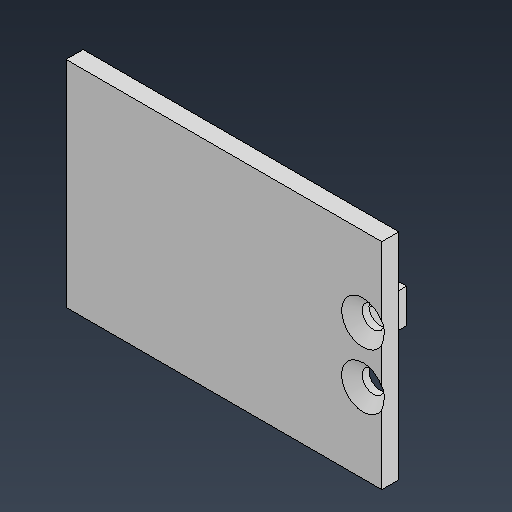
# Autodesk Inventor part: PCB_Holder_Floor
Saved by Autodesk Inventor 2026.2 (Build 302298010, 298A)
## iProperties
Created: 2026-04-05
Part Number: PCB_Holder_Floor
Material: Generic
Document SubType Name: Modeling
Designer: szymo
Density: 1 g/cm^3
Appearance: Default
Author: szymo
Autodesk Inventor part; units mm, degrees
ref_plane "YZ Plane" through (0, 0, 0) normal (1, 0, 0) x (0, 1, 0)
ref_plane "XZ Plane" through (0, 0, 0) normal (0, 1, 0) x (-1, 0, 0)
ref_plane "XY Plane" through (0, 0, 0) normal (0, 0, 1) x (1, 0, 0)
sketch "Sketch1" plane through (0, 0, 0) normal (0, 0, 1) x (1, 0, 0)
  line L0 (-1.35, 35.9569) -> (-38.25, 35.9569)
  line L1 (-38.25, 35.9569) -> (-38.25, 22.861)
  line L2 (-38.25, 22.861) -> (-1.35, 22.861)
  line L3 (-1.35, 22.861) -> (-1.35, 35.9569)
  line L4 (-5.95, 27.409) -> (-11.45, 27.409)
  line L5 (-11.45, 27.409) -> (-11.45, 31.409)
  line L6 (-11.45, 31.409) -> (-5.95, 31.409)
  line L7 (-5.95, 31.409) -> (-5.95, 27.409)
  line L8 (-28.15, 27.409) -> (-33.65, 27.409)
  line L9 (-33.65, 27.409) -> (-33.65, 31.409)
  line L10 (-33.65, 31.409) -> (-28.15, 31.409)
  line L11 (-28.15, 31.409) -> (-28.15, 27.409)
  line L12 (-1.35, 22.861) -> (-1.35, 16.861)
  line L13 (-1.35, 16.861) -> (-38.25, 16.861)
  line L14 (-38.25, 16.861) -> (-38.25, 22.861)
  line L15 (-38.25, 35.9569) -> (-38.25, 41.9569)
  line L16 (-38.25, 41.9569) -> (-1.35, 41.9569)
  line L17 (-1.35, 41.9569) -> (-1.35, 35.9569)
  line L18 (-1.35, 22.861) -> (-5.55, 22.861) projected
  line L19 (-1.35, 35.9569) -> (-1.35, 22.861) projected
  line L20 (-1.35, 35.9569) -> (-5.15, 35.9569) projected
  line L21 (-38.25, 37.1263) -> (-38.25, 24.4355) projected
  line L22 (-38.25, 24.4355) -> (-34.05, 24.4355) projected
  circle A0 centre (-3.55, 32.6677) radius 2 projected
  circle A1 centre (-3.55, 32.6677) radius 2 projected
  circle A2 centre (-3.55, 26.1197) radius 2 projected
  circle A3 centre (-3.55, 26.1197) radius 2 projected
  line L23 (-5.15, 35.2466) -> (-5.15, 35.9569) projected
  line L24 (-5.15, 35.2466) -> (-5.55, 35.2466) projected
  line L25 (-5.55, 32.6677) -> (-5.55, 35.2466) projected
  line L26 (-5.55, 26.1197) -> (-5.55, 32.6677) projected
  line L27 (-5.55, 22.861) -> (-5.55, 26.1197) projected
  line L28 (-34.05, 37.1263) -> (-34.05, 24.4355) projected
  line L29 (-38.25, 37.1263) -> (-34.05, 37.1263) projected
  ellipse E0 centre (-36.15, 27.6082) end of major axis (-38.15, 27.6082) minor radius 1.9381 projected
  ellipse E1 centre (-36.15, 33.9536) end of major axis (-38.15, 33.9536) minor radius 1.9381 projected
  point P0 (0, 0)
  point P1 (-3.45, 33.6719)
  point P2 (-3.45, 27.124)
  point P3 (-34.55, 27.124)
  point P4 (-34.55, 33.6719)
  point P5 (-4.75, 22.861)
  point P6 (-33.25, 32.7932)
  point P7 (-36.65, 32.7932)
  point P8 (-33.85, 22.832)
  point P9 (-8.7, 31.409)
  point P10 (-34.85, 35.9278)
  dimension "d1" = 5.5
  dimension "d23" = 6
  dimension "d24" = 6
  dimension "d25" = 0
  dimension "d26" = 0
  dimension "d27" = 0
  dimension "d28" = 0
  dimension "d29" = 5.5
  dimension "d33" = 4
  dimension "d34" = 4
  dimension "d35" = 4.5479
  dimension "d36" = 4.5479
  dimension "d37" = 4.5479
  dimension "d38" = 4.5479
  constraints: 32 end point, 5 parallel, 4 perpendicular, 3 horizontal, 3 vertical, 2 horizontal alignment, 1 midpoint, 1 point on line, 9 other
  measures "d1" distance between parallel lines of L7 L5
  measures "d25" distance between parallel lines of L1 L21
  measures "d26" distance between parallel lines of L3 L19
  measures "d27" vertical extent of L20
  measures "d28" vertical extent of L18
  measures "d29" distance between parallel lines of L11 L9
  measures "d33" distance of L4.end L5.end
  measures "d34" distance of L10.end L8.start
extrude "Extrusion1" add sketch "Sketch1" against normal blind 2 contours A0 | A2 | L3 L2 L27 L26 L25 L24 L23 L0 | L0 L28 L29 L15 L16 L17 | L23 L24 L25 L26 L27 L2 L1 L22 L28 L0 | L12 L13 L14 L2 | L28 L22 L1 L0 | L0 L15 L29 L28 | L4 L5 L6 L7 | L8 L9 L10 L11 | E0 | E1
extrude "Extrusion2" add sketch "Sketch1" against normal blind 7.5 contours L4 L5 L6 L7 | L8 L9 L10 L11
sketch "Sketch2" plane through (-11.8, 27.409, -2) normal (0, -1, 0) x (1, 0, 0)
  line L0 (5.85, -5.5) -> (0.175, 0.175)
  line L1 (0.35, -5.5) -> (5.85, 0)
  line L2 (-16.35, -5.5) -> (-21.85, 0)
  line L3 (-21.85, -5.5) -> (-16.35, 0)
  circle A0 centre (3.1, -2.75) radius 2.75
  circle A1 centre (-19.1, -2.75) radius 2.75
  line L4 (5.85, 0) -> (5.85, -5.5) projected
  line L5 (-21.85, 0) -> (-21.85, -5.5) projected
  line L6 (0.35, -5.5) -> (5.85, -5.5) projected
  line L7 (5.85, -5.5) -> (0.35, -5.5)
  line L8 (-21.85, -5.5) -> (-16.35, -5.5) projected
  line L9 (-21.85, -5.5) -> (-16.35, -5.5)
  point P0 (11.8, 2)
  point P1 (5.85, 2)
  dimension "d13" = 5.5
  dimension "d14" = 5.5
  constraints: 12 end point, 3 midpoint, 3 point on line, 2 centre point, 2 coincident, 2 collinear, 2 parallel, 1 perpendicular
  measures "d13" diameter of A0
  measures "d14" diameter of A1
hole "Hole1" at (-8.7, 27.409, -4.75) at (-30.9, 27.409, -4.75) direction (0, 1, 0) diameter 2.5 end through all
fillet "Fillet1" radius 1 2 edges at (-11.45, 29.409, -7.5) (-28.15, 29.409, -7.5)
hole "Hole2" at (-3.55, 32.6677, 0) at (-3.55, 26.1197, 0) direction (0, 0, -1) diameter 2.6 end through all countersink diameter 5 countersink angle 90 clearance for "Countersunk Flat Head Screw ISO 2009/7046" size "M2" standard "ISO"
equation "\"d23\" = d24"
equation "\"d29\" = d1"
body "Solid1"
